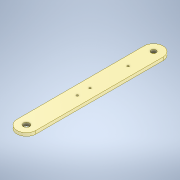
# Autodesk Inventor part: Canh_Tay_1
Saved by Autodesk Inventor 2022 (Build 260153000, 153)
## iProperties
Created: 2022-11-10
Part Number: Canh_Tay_1
Material: Nylon 6/6
Document SubType Name: Modeling
Designer: nguye
Density: 1.13 g/cm^3
Appearance: Nylon 6
Author: nguye
Autodesk Inventor part; units mm, degrees
ref_plane "YZ Plane" through (0, 0, 0) normal (1, 0, 0) x (0, 1, 0)
ref_plane "XZ Plane" through (0, 0, 0) normal (0, 1, 0) x (-1, 0, 0)
ref_plane "XY Plane" through (0, 0, 0) normal (0, 0, 1) x (1, 0, 0)
sketch "Sketch1" plane through (0, 0, 0) normal (0, 1, 0) x (-1, 0, 0)
  circle A0 centre (0, 0) radius 4
  circle A1 centre (0, 200) radius 15
  circle A2 centre (0, 200) radius 5
  circle A3 centre (0, 0) radius 15
  line L0 (15, 200) -> (15, 0)
  line L1 (-15, 200) -> (-15, 0)
  line L2 (0, 160) -> (0, 110) construction
  line L3 (4, 160) -> (4, 110)
  line L4 (-4, 110) -> (-4, 160)
  arc A4 (4, 160) -> (-4, 160) centre (0, 160) ccw
  arc A5 (-4, 110) -> (4, 110) centre (0, 110) ccw
  line L5 (0, -61) -> (0, 261) projected
  line L6 (4, 90) -> (4, 40)
  arc A6 (4, 90) -> (-4, 90) centre (0, 90) ccw
  line L7 (-4, 40) -> (-4, 90)
  arc A7 (-4, 40) -> (4, 40) centre (0, 40) ccw
  circle A8 centre (0, 175) radius 1.5
  circle A9 centre (0, 100) radius 1.5
  circle A10 centre (0, 120) radius 1.5
  circle A11 centre (0, 40) radius 1.5
  point P0 (0, 135)
  point P1 (-7, 0)
  point P2 (7, 0)
  point P3 (0, 121.5)
  point P4 (0, 118.5)
  dimension "d0" = 8
  dimension "d1" = 30
  dimension "d2" = 200
  dimension "d3" = 10
  dimension "d4" = 30
  dimension "d16" = 8
  dimension "d18" = 50
  dimension "d20" = 14
  dimension "d21" = 7
  dimension "d31" = 65
  dimension "d34" = 70
  dimension "d39" = 40
  dimension "d40" = 40
  dimension "d41" = 75
  dimension "d44" = 3
  dimension "d45" = 3
  dimension "d46" = 3
  dimension "d47" = 25
  dimension "d48" = 3
  dimension "d50" = 40
  dimension "d51" = 100
  dimension "d52" = 120
  constraints: 16 end point, 12 centre point, 12 point on circle, 7 tangent, 6 coincident, 3 vertical, 3 vertical alignment, 2 horizontal alignment, 2 midpoint, 2 point on line, 1 parallel, 10 other
  measures "d0" diameter of A0
  measures "d1" diameter of A1
  measures "d2" distance of point (0, 0) A1.centre
  measures "d3" diameter of A2
  measures "d4" diameter of A3
  measures "d16" distance between parallel lines of L4 L3
  measures "d18" distance of L2.end L2.start
  measures "d20" distance of point (7, 0) point (-7, 0)
  measures "d21" distance of A0.centre point (-7, 0)
  measures "d31" distance of A1.centre point (0, 135)
  measures "d34" distance of L3.start L6.start
  measures "d39" distance of L2.start A1.centre
  measures "d40" distance of point (0, 0) A7.centre
  measures "d41" distance of point (0, 100) point (0, 175)
  measures "d44" diameter of A8
  measures "d45" diameter of A9
  measures "d46" diameter of A10
  measures "d47" distance of A2.centre A8.centre
  measures "d48" diameter of A11
  measures "d50" distance of point (0, 0) A11.centre
  measures "d51" distance of point (0, 0) A9.centre
  measures "d52" distance of point (0, 0) A10.centre
extrude "Extrusion1" add sketch "Sketch1" along normal blind 5 contours A0 L5 A3 | A0 L5 A3 | L5 A7 L6 A6 A9 A5 L3 A4 A8 A1 L0 A3 | A3 L1 A1 L5 A8 A4 L4 A5 A9 A6 L7 A7 | A7 L7 A6 L5 A11 | L5 A11 A6 L6 A7 | A1 L5 A2 | A1 L5 A2 | A8 L5 | L5 A8 | L5 A10 A5 L4 A4 | A4 L3 A5 L5 A10
body "Solid1"
